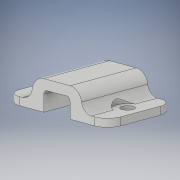
# Autodesk Inventor part: small-cable-clip
Saved by Autodesk Inventor 2018 (Build 220112000, 112)
## iProperties
Created: 2020-01-09
Part Number: small-cable-clip
Material: Generic
Document SubType Name: Modeling
Designer: Vinnie Caprarola
Density: 1 g/cm^3
Appearance: Default
Author: Vinnie Caprarola
Autodesk Inventor part; units mm, degrees
ref_plane "YZ Plane" through (0, 0, 0) normal (1, 0, 0) x (0, 1, 0)
ref_plane "XZ Plane" through (0, 0, 0) normal (0, 1, 0) x (-1, 0, 0)
ref_plane "XY Plane" through (0, 0, 0) normal (0, 0, 1) x (1, 0, 0)
sketch "Sketch1" plane through (0, 0, 0) normal (0, 0, 1) x (1, 0, 0)
  line L0 (0, 0) -> (8, 0)
  line L1 (8, 0) -> (8, 3.5)
  line L2 (8, 3.5) -> (0, 3.5)
  line L3 (0, 3.5) -> (0, 0)
  line L4 (0, 7) -> (8, 7)
  arc A0 (11.5, 3.5) -> (8, 7) centre (8, 3.5) ccw
  line L5 (11.5, 3.5) -> (11.5, -3.5)
  line L6 (11.5, -3.5) -> (-3.5, -3.5)
  line L7 (-3.5, -3.5) -> (-3.5, 3.5)
  arc A1 (0, 7) -> (-3.5, 3.5) centre (0, 3.5) ccw
  line L8 (0, 0) -> (0, -3.5)
  line L9 (8, 0) -> (8, -3.5)
  line L10 (-3.5, -3.5) -> (-11.5, -3.5)
  line L11 (-11.5, -3.5) -> (-11.5, -1.5)
  line L12 (-11.5, -1.5) -> (-3.5, -1.5)
  line L13 (-3.5, -1.5) -> (-3.5, -3.5)
  line L14 (11.5, -3.5) -> (19.5, -3.5)
  line L15 (19.5, -3.5) -> (19.5, -1.5)
  line L16 (19.5, -1.5) -> (11.5, -1.5)
  line L17 (11.5, -1.5) -> (11.5, -3.5)
  point P0 (8, 3.5)
  point P1 (0, 3.5)
  dimension "d2" = 0
  dimension "d0" = 8
  dimension "d1" = 3.5
  dimension "d3" = 3.5
  dimension "d6" = 8
  dimension "d7" = 2
  dimension "d8" = 8
  dimension "d9" = 2
  constraints: 36 end point, 9 parallel, 6 point on line, 5 horizontal, 5 perpendicular, 4 point on circle, 2 centre point, 2 vertical, 13 other
  measures "d0" distance of point (0, 3.5) point (8, 3.5)
  measures "d1" distance of point (8, 3.5) L0.end
  measures "d3" distance between parallel lines of L2 L4
  measures "d6" distance of L11.end L12.end
  measures "d7" distance of L10.end L11.end
  measures "d8" distance of L16.end L15.end
  measures "d9" distance of L15.end L14.end
extrude "Extrusion2" add sketch "Sketch1" along normal blind 20 contours L8 L6 L7 A1 L4 A0 L5 L9 L1 L2 L3 | L10 L11 L12 L7 | L5 L16 L15 L14
fillet "Fillet1" radius 3 2 edges at (11.5, -1.5, 10) (-3.5, -1.5, 10)
fillet "Fillet3" radius 4 4 edges at (-11.5, -2.5, 20) (-11.5, -2.5, 0) (19.5, -2.5, 20) (19.5, -2.5, 0)
sketch "Sketch2" plane through (14.5, -1.5, 20) normal (0, 1, 0) x (1, 0, 0)
  circle A0 centre (1, 10) radius 1.75
  line L0 (5, 16) -> (5, 4) projected
  circle A1 centre (1, 10) radius 3.5
  line L1 (-6.5, 20) -> (-14.5, 20) projected
  line L2 (-10.5, 20) -> (-10.5, 23.3018)
  circle A2 centre (-22, 10) radius 1.75
  circle A3 centre (-22, 10) radius 3.5
  point P0 (-14.5, 20)
  point P1 (5, 10)
  dimension "d16" = 4
  dimension "d17" = 3.5
  dimension "d18" = 7
  constraints: 4 centre point, 2 coincident, 2 end point, 2 midpoint, 2 symmetric about line, 1 horizontal alignment, 1 vertical, 2 other
  measures "d16" distance from line of A0.centre L0
  measures "d17" diameter of A0
  measures "d18" diameter of A1
extrude "Extrusion3" cut sketch "Sketch2" against normal through all contours A0 | A2
extrude "Extrusion4" cut sketch "Sketch2" along normal through all contours A0 | A1 | A2 | A3
thicken "Thicken2" operation add thickness 1 both sides no extend neighbours yes toward (0, -1, 0) faces at (5.3333, 7, 6.6667)
thicken "Thicken3" operation add thickness 2 both sides no extend neighbours yes toward (0, -1, 0) faces at (2.6667, 3.5, 6.6667)
thicken "Thicken4" operation add thickness 2 both sides no extend neighbours yes toward (0, -1, 0) faces at (5.3333, 6, 6.6667)
fillet "Fillet4" radius 1 2 edges at (0, 1.5, 10) (8, 1.5, 10)
body "Solid2"
